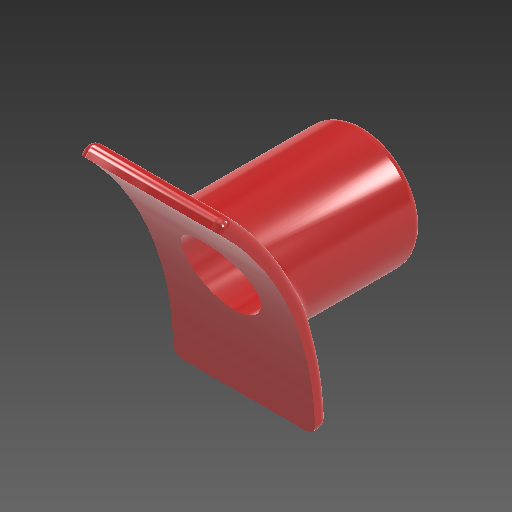
# Autodesk Inventor part: strut_flange
Saved by Autodesk Inventor 2020.2 (Build 242310000, 310)
## iProperties
Created: 2020-03-22
Part Number: strut_flange
Material: Wood (Birch)
Document SubType Name: Modeling
Designer: agmle
Density: 0.55 g/cm^3
Appearance: Red
Mass: 29.7525 g
Surface Area: 195.167 cm^2
Volume: 54.0954 cm^3
strut_hole_offset: 1.646 in
Author: agmle
Autodesk Inventor part; units mm, degrees
ref_plane "YZ Plane" through (0, 0, 0) normal (1, 0, 0) x (0, 1, 0)
ref_plane "XZ Plane" through (0, 0, 0) normal (0, 1, 0) x (-1, 0, 0)
sketch "Sketch1" plane through (0, 0, 0) normal (1, 0, 0) x (0, 1, 0)
  arc A0 (0, -114.5375) -> (83.6335, -78.2578) centre (0, 0) ccw
  arc A1 (0, -109.5375) -> (79.9826, -74.8415) centre (0, 0) ccw
  line L0 (79.9826, -74.8415) -> (83.6335, -78.2578)
  line L1 (0, -114.5375) -> (0, -109.5375)
  line L2 (63.0122, -109.5375) -> (33.472, -109.5375) construction
  line L3 (33.472, -109.5375) -> (33.472, -399.3065) construction
  line L4 (33.472, -399.3065) -> (63.0122, -399.3065) construction
  line L5 (63.0122, -399.3065) -> (63.0122, -109.5375) construction
  circle A2 centre (0, 0) radius 109.5375 construction
  line L6 (0, 0) -> (33.472, -109.5375) construction
  line L7 (0, 0) -> (63.0122, -109.5375) construction
  line L8 (0, -112.0375) -> (33.472, -109.5375) construction
  line L9 (81.808, -76.5497) -> (57.1128, -99.2823) construction
  dimension "d0" = 5
  dimension "d1" = 109.5375
  dimension "d2" = 29.5402
  constraints: 20 end point, 6 point on circle, 4 coincident, 3 centre point, 2 line through centre, 2 midpoint, 2 parallel, 1 concentric, 1 equal length, 1 horizontal, 1 perpendicular, 1 point on line, 1 tangent, 1 vertical
  measures "d0" distance of L1.start L1.end
  measures "d1" radius of A1
  measures "d2" distance of L2.start L2.end
extrude "Flange" add sketch "Sketch1" along normal blind 50.8
ref_plane "Work Plane1" through (0, 0, -114.5375) normal (0, 0, 1) x (1, 0, 0)
sketch "Sketch2" plane through (0, 0, -114.5375) normal (0, 0, 1) x (1, 0, 0)
  line L0 (0, 83.6335) -> (50.8, 83.6335) construction
  line L1 (25.4, 83.6335) -> (25.4, 0) construction
  line L2 (0, 0) -> (50.8, 0) construction
  circle A0 centre (25.4, 41.8167) radius 21.1201
  line L3 (0, 79.9826) -> (0, 0) construction
  dimension "d18" = 42.2402
  constraints: 3 midpoint, 2 end point, 1 centre point, 1 coincident
  measures "d18" diameter of A0
extrude "Mount Part A" add sketch "Sketch2" along normal up to next
sketch "Sketch3" plane through (25.4, 41.8167, -114.5375) normal (0, 0, -1) x (-1, 0, 0)
  circle A0 centre (0, 0) radius 21.1201 projected
  point P0 (25.4, -41.8167)
extrude "Mount Part B" add sketch "Sketch3" along normal blind 38.1
sketch "Sketch4" plane through (25.4, 41.8167, -152.6375) normal (0, 0, -1) x (-1, 0, 0)
  circle A0 centre (0, 0) radius 21.1201 projected
  point P0 (25.4, -41.8167)
  constraints: 2 coincident
hole "EMT Bore" at (25.4, 41.8167, -152.6375) direction (0, 0, 1) diameter 26.6446 end through all counterbore diameter 29.5402 counterbore depth 38.1
fillet "Softening" radius 3.175 11 edges at (4.3481, 43.513, -105.9503) (0, 0, -112.0375) (50.8, 0, -112.0375) (0, 81.808, -76.5497) (50.8, 81.808, -76.5497) (46.5201, 41.8167, -152.6375) (25.4, 27.0466, -152.6375) (50.8, 45.5817, -105.0769) (25.4, 0, -114.5375) (0, 45.5817, -105.0769) (25.4, 83.6335, -78.2578)
sketch "Sketch5" plane through (0, 0, 0) normal (1, 0, 0) x (0, 1, 0)
  arc A0 (3.175, -109.4915) -> (77.7796, -77.1284) centre (0, 0) ccw construction
  line L0 (27.0466, -114.5375) -> (56.5868, -114.5375) construction
  line L1 (56.5868, -149.4625) -> (27.0466, -149.4625) construction
  point P0 (41.8167, -114.5375)
  dimension "strut_hole_offset" = 41.8167
  constraints: 1 midpoint
  measures "strut_hole_offset" horizontal distance of A0.centre point (41.817, -114.537)
equation "\"d1\" = 0.5 * hull_od"
equation "\"d2\" = conduit_od"
equation "\"d10\" = conduit_od - 2 * conduit_wall_thick"
equation "\"d12\" = conduit_od"
equation "\"hull_od\" = 219.075"
equation "\"hull_id\" = 201.7268"
equation "\"hull_wall\" = 8.6741"
equation "\"hull_length\" = 609.6"
equation "\"hull_spacing\" = 390.525"
equation "\"impeller_od\" = 76.2"
equation "\"impeller_clearance\" = 0.5"
equation "\"impeller_shaft_id\" = 3.175"
equation "\"impeller_shaft_od\" = 5.715"
equation "\"impeller_shaft_support\" = 3.175"
equation "\"impeller_intake_od\" = 19.05"
equation "\"impeller_vane_thick\" = 2"
equation "\"impeller_vane_inner_rad\" = 3.175"
equation "\"impeller_vane_outer_rad\" = 0.37206"
equation "\"magnet_od\" = 5.95"
equation "\"magnet_clearance\" = 0.25"
equation "\"magnet_rad\" = 0.25"
equation "\"magnet_circle_offset\" = 3.175"
equation "\"motor_shaft_od\" = 12.7"
equation "\"motor_shaft_length\" = 31.75"
equation "\"motor_shaft_key\" = 3.048"
equation "\"slab_thick\" = 34.671"
equation "\"conduit_od\" = 29.5402"
equation "\"conduit_wall_thick\" = 1.4478"
body "Solid1"
